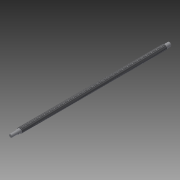
# Autodesk Inventor part: ZACMEScrew
Saved by Autodesk Inventor 2015 (Build 190159000, 159)
## iProperties
Created: 2014-01-02
Part Number: ZACMEScrew
Material: Steel
Document SubType Name: Modeling
Designer: Jack
Density: 7.85 g/cm^3
Appearance: Steel
Author: Jack
Autodesk Inventor part; units mm, degrees
ref_plane "YZ Plane" through (0, 0, 0) normal (1, 0, 0) x (0, 1, 0)
ref_plane "XZ Plane" through (0, 0, 0) normal (0, 1, 0) x (-1, 0, 0)
ref_plane "XY Plane" through (0, 0, 0) normal (0, 0, 1) x (1, 0, 0)
sketch "Sketch1" plane through (0, 0, 0) normal (0, 1, 0) x (-1, 0, 0)
  circle A0 centre (0, 0) radius 3.15
  dimension "d0" = 6.3
  constraints: 1 centre point, 1 coincident
  measures "d0" diameter of A0
extrude "Extrusion1" add sketch "Sketch1" along normal blind 12
sketch "Sketch2" plane through (0, 12, 0) normal (0, 1, 0) x (1, 0, 0)
  circle A0 centre (0, 0) radius 3.15 projected
  circle A1 centre (0, 0) radius 3.9
  dimension "d3" = 7.8
  constraints: 1 centre point, 1 coincident
  measures "d3" diameter of A1
extrude "Extrusion2" add sketch "Sketch2" along normal blind 6 contours A0 | A1
chamfer "Chamfer1" distance 0.75 angle 45 1 edges at (-3.9, 12, 0)
sketch "Sketch3" plane through (0, 18, 0) normal (0, 1, 0) x (1, 0, 0)
  circle A0 centre (0, 0) radius 3.9 projected
  circle A1 centre (0, 0) radius 5
  dimension "d9" = 10
  constraints: 1 centre point, 1 coincident
  measures "d9" diameter of A1
extrude "Extrusion3" add sketch "Sketch3" along normal blind 286 contours A0 | A1
sketch "Sketch4" plane through (0, 304, 0) normal (0, 1, 0) x (1, 0, 0)
  circle A0 centre (0, 0) radius 5 projected
  circle A1 centre (0, 0) radius 3.9
  dimension "d12" = 7.8
  constraints: 1 centre point, 1 coincident
  measures "d12" diameter of A1
extrude "Extrusion4" add sketch "Sketch4" along normal blind 10 contours A1
chamfer "Chamfer2" distance 0.5 angle 45 2 edges at (-3.9, 314, 0) (3.15, 0, 0)
thread "Thread1" size "TR10x2" class "7e" standard "ISO Metric Trapezoidal Threads" full length
body "Solid1"
